Autodesk Fusion 360 part; units mm, degrees
(part 5 of 5)
sketch "Sketch2" plane through (0, 0, 2) normal (0, 0, 1) x (1, 0, 0)
  arc A0 (20.1662, -102.4349) -> (20.2, -101.6132) centre (10.2, -101.6132) ccw
  line L0 (20.2, -101.6132) -> (20.2, -87.2749)
  arc A1 (22.987, -85.4363) -> (20.2, -87.2749) centre (22.2, -87.2749) ccw
  line L1 (22.987, -85.4363) -> (27.3521, -87.3046)
  arc A2 (27.3521, -87.3046) -> (36.4601, -74.6136) centre (30.5, -79.95) ccw
  line L2 (36.4601, -74.6136) -> (31.6483, -69.2394)
  arc A3 (29.5877, -66.4969) -> (31.6483, -69.2394) centre (46.5487, -55.8985) ccw
  line L3 (29.5877, -66.4969) -> (23.2215, -56.3087)
  arc A4 (21.55, -50.4796) -> (23.2215, -56.3087) centre (32.55, -50.4796) ccw
  line L4 (21.55, -50.4796) -> (21.55, -18.7607)
  arc A5 (23.2215, -12.9316) -> (21.55, -18.7607) centre (32.55, -18.7607) ccw
  line L5 (23.2215, -12.9316) -> (27.7114, -5.7461)
  arc A6 (33.9547, -0.1656) -> (27.7114, -5.7461) centre (40.4322, -13.6949) ccw
  arc A7 (33.9547, -0.1656) -> (30.5, 15.05) centre (30.5, 7.05) ccw
  line L6 (30.5, 15.05) -> (9.313, 15.05)
  arc A8 (5, 18) -> (9.313, 15.05) centre (9.313, 19.6778) ccw
  line L7 (5, 18) -> (-5, 18)
  arc A9 (-9.313, 15.05) -> (-5, 18) centre (-9.313, 19.6778) ccw
  line L8 (-9.313, 15.05) -> (-30.5, 15.05)
  arc A10 (-30.5, 15.05) -> (-33.9547, -0.1656) centre (-30.5, 7.05) ccw
  arc A11 (-27.7114, -5.7461) -> (-33.9547, -0.1656) centre (-40.4322, -13.6949) ccw
  line L9 (-27.7114, -5.7461) -> (-23.2215, -12.9316)
  arc A12 (-21.55, -18.7607) -> (-23.2215, -12.9316) centre (-32.55, -18.7607) ccw
  line L10 (-21.55, -18.7607) -> (-21.55, -50.4796)
  arc A13 (-23.2215, -56.3087) -> (-21.55, -50.4796) centre (-32.55, -50.4796) ccw
  line L11 (-23.2215, -56.3087) -> (-29.5877, -66.4969)
  arc A14 (-31.6483, -69.2394) -> (-29.5877, -66.4969) centre (-46.5487, -55.8985) ccw
  line L12 (-31.6483, -69.2394) -> (-36.4601, -74.6136)
  arc A15 (-36.4601, -74.6136) -> (-27.3521, -87.3046) centre (-30.5, -79.95) ccw
  line L13 (-27.3521, -87.3046) -> (-22.987, -85.4363)
  arc A16 (-20.2, -87.2749) -> (-22.987, -85.4363) centre (-22.2, -87.2749) ccw
  line L14 (-20.2, -87.2749) -> (-20.2, -101.6132)
  arc A17 (-20.2, -101.6132) -> (-20.1662, -102.4349) centre (-10.2, -101.6132) ccw
  line L15 (-20.1662, -102.4349) -> (-19.6835, -108.2886)
  arc A18 (-19.6835, -108.2886) -> (-19.1143, -110.8871) centre (-9.7173, -107.4669) ccw
  line L16 (-19.1143, -110.8871) -> (-15.7286, -120.1891)
  arc A19 (-15.7286, -120.1891) -> (-7.0571, -119.3647) centre (-11.5, -118.65) ccw
  arc A20 (-3.1079, -116) -> (-7.0571, -119.3647) centre (-3.1079, -120) ccw
  line L17 (-3.1079, -116) -> (3.1079, -116)
  arc A21 (7.0571, -119.3647) -> (3.1079, -116) centre (3.1079, -120) ccw
  arc A22 (7.0571, -119.3647) -> (15.7286, -120.1891) centre (11.5, -118.65) ccw
  line L18 (15.7286, -120.1891) -> (19.1143, -110.8871)
  arc A23 (19.1143, -110.8871) -> (19.6835, -108.2886) centre (9.7173, -107.4669) ccw
  line L19 (19.6835, -108.2886) -> (20.1662, -102.4349)
  circle A24 centre (-15.25, -49.85) radius 1.5
  arc A25 (-13.5, 3) -> (-15.1961, -0.0598) centre (-13.5, 1) ccw
  line L20 (-13.5, 3) -> (-10.3384, 3)
  arc A26 (-6.0958, 1.2426) -> (-10.3384, 3) centre (-10.3384, -3) ccw
  line L21 (-6.0958, 1.2426) -> (-4.8532, 0)
  line L22 (-4.8532, 0) -> (4.8532, 0)
  line L23 (4.8532, 0) -> (6.0958, 1.2426)
  arc A27 (10.3384, 3) -> (6.0958, 1.2426) centre (10.3384, -3) ccw
  line L24 (10.3384, 3) -> (13.5, 3)
  arc A28 (15.1961, -0.0598) -> (13.5, 3) centre (13.5, 1) ccw
  line L25 (15.1961, -0.0598) -> (9.0119, -10.0491)
  spline S0 degree 5 poles (9.0119, -10.0491) (8.9382, -10.1683) (8.7794, -10.3902) (8.5077, -10.6735) (8.0875, -10.964) (7.4965, -11.2156) (6.9894, -11.3405) (6.5947, -11.3892) (6.3253, -11.4) (6.189, -11.4) knots 0 0 0 0 0 0 0.2 0.4 0.6 0.8 1 1 1 1 1 1
  line L26 (6.189, -11.4) -> (-6.189, -11.4)
  spline S1 degree 5 poles (-6.189, -11.4) (-6.3253, -11.4) (-6.5947, -11.3892) (-6.9894, -11.3405) (-7.4965, -11.2156) (-8.0875, -10.964) (-8.5077, -10.6735) (-8.7794, -10.3902) (-8.9382, -10.1683) (-9.0119, -10.0491) knots -1 -1 -1 -1 -1 -1 -0.8 -0.6 -0.4 -0.2 0 0 0 0 0 0
  line L27 (-9.0119, -10.0491) -> (-15.1961, -0.0598)
  circle A29 centre (15.25, -49.85) radius 1.5
  circle A30 centre (15.25, -19.35) radius 1.5
  circle A31 centre (-15.25, -19.35) radius 1.5
  circle A32 centre (-15.25, -63.85) radius 1.5
  circle A33 centre (-30.5, 7.05) radius 3.375
  circle A34 centre (15, -73.65) radius 1.5
  circle A35 centre (-15, -73.65) radius 1.5
  circle A36 centre (-10, -44.6) radius 1.5
  circle A37 centre (10, -44.6) radius 1.5
  circle A38 centre (10, -24.6) radius 1.5
  circle A39 centre (-10, -24.6) radius 1.5
  line L28 (5.45, -24.029) -> (5.45, -45.171)
  arc A40 (5.2981, -46.9075) -> (5.45, -45.171) centre (-4.55, -45.171) ccw
  line L29 (5.2981, -46.9075) -> (4.4577, -51.6736)
  arc A41 (3.4729, -52.5) -> (4.4577, -51.6736) centre (3.4729, -51.5) ccw
  line L30 (3.4729, -52.5) -> (-3.4729, -52.5)
  arc A42 (-4.4577, -51.6736) -> (-3.4729, -52.5) centre (-3.4729, -51.5) ccw
  line L31 (-4.4577, -51.6736) -> (-5.2981, -46.9075)
  arc A43 (-5.45, -45.171) -> (-5.2981, -46.9075) centre (4.55, -45.171) ccw
  line L32 (-5.45, -45.171) -> (-5.45, -24.029)
  arc A44 (-5.2981, -22.2925) -> (-5.45, -24.029) centre (4.55, -24.029) ccw
  line L33 (-5.2981, -22.2925) -> (-4.4577, -17.5264)
  arc A45 (-3.4729, -16.7) -> (-4.4577, -17.5264) centre (-3.4729, -17.7) ccw
  line L34 (-3.4729, -16.7) -> (3.4729, -16.7)
  arc A46 (4.4577, -17.5264) -> (3.4729, -16.7) centre (3.4729, -17.7) ccw
  line L35 (4.4577, -17.5264) -> (5.2981, -22.2925)
  arc A47 (5.45, -24.029) -> (5.2981, -22.2925) centre (-4.55, -24.029) ccw
  circle A48 centre (30.5, 7.05) radius 3.375
  circle A49 centre (-30.5, -79.95) radius 3.375
  circle A50 centre (15.25, -63.85) radius 1.5
  circle A51 centre (15.25, 8.95) radius 1.5
  circle A52 centre (-15.25, 8.95) radius 1.5
  arc A53 (4.5, -61) -> (8.3897, -57.7389) centre (6.3028, -59.2001) ccw
  line L36 (4.5, -61) -> (-4.5, -61)
  arc A54 (-8.3897, -57.7389) -> (-4.5, -61) centre (-6.3028, -59.2001) ccw
  line L37 (-8.3897, -57.7389) -> (-8.0447, -57.2462)
  arc A55 (-6.6112, -56.5) -> (-8.0447, -57.2462) centre (-6.6112, -58.25) ccw
  line L38 (-6.6112, -56.5) -> (6.6112, -56.5)
  arc A56 (8.0447, -57.2462) -> (6.6112, -56.5) centre (6.6112, -58.25) ccw
  line L39 (8.0447, -57.2462) -> (8.3897, -57.7389)
  circle A57 centre (30.5, -79.95) radius 3.375
  circle A58 centre (11.5, -118.65) radius 1.5
  circle A59 centre (15, -103.65) radius 1.5
  circle A60 centre (-11.5, -118.65) radius 1.5
  circle A61 centre (-15, -103.65) radius 1.5
  line L40 (0, -116) -> (0, -61) construction
  line L41 (-15, -103.65) -> (-5.1101, -103.65) construction
  circle A62 centre (-10, -103.65) radius 1
  circle A63 centre (-10, -103.65) radius 3
  line L42 (-2.5, -103.3105) -> (-2.5, -113.346)
  line L43 (-2.5, -113.346) -> (-11.1856, -107.81)
  line L44 (-11.1856, -107.81) -> (-11.1856, -106.4058)
  line L45 (-2.5, -103.3105) -> (-4.5464, -101.7117)
  line L46 (-7, -103.65) -> (-7, -103.4617)
  line L47 (-5.25, -101.7117) -> (-4.5464, -101.7117)
  arc A64 (-5.25, -101.7117) -> (-7, -103.4617) centre (-5.25, -103.4617) ccw
  line L48 (-10, -103.65) -> (-10, -83.65) construction
  circle A65 centre (-10, -83.65) radius 1
  circle A66 centre (-10, -83.65) radius 3
  line L49 (-2.5, -84.401) -> (-2.5, -94.9628)
  line L50 (-2.5, -84.401) -> (-5.6804, -81.9162)
  line L51 (-2.5, -84.401) -> (1.142, -84.401) construction
  line L52 (-5.6804, -81.9162) -> (-7.3512, -85.0584)
  line L53 (-9.532, -86.6133) -> (-9.532, -90.422)
  line L54 (-9.532, -90.422) -> (-2.5, -94.9628)
  line L55 (10, -103.65) -> (10, -83.65) construction
  line L56 (2.5, -103.3105) -> (4.5464, -101.7117)
  line L57 (2.5, -103.3105) -> (2.5, -113.346)
  circle A67 centre (10, -103.65) radius 3
  line L58 (2.5, -113.346) -> (11.1856, -107.81)
  circle A68 centre (15, -103.65) radius 1.5
  line L59 (15, -103.65) -> (5.1101, -103.65) construction
  line L60 (11.1856, -107.81) -> (11.1856, -106.4058)
  line L61 (7, -103.65) -> (7, -103.4617)
  circle A69 centre (10, -103.65) radius 1
  line L62 (5.25, -101.7117) -> (4.5464, -101.7117)
  arc A70 (7, -103.4617) -> (5.25, -101.7117) centre (5.25, -103.4617) ccw
  line L63 (9.532, -90.422) -> (2.5, -94.9628)
  line L64 (2.5, -84.401) -> (2.5, -94.9628)
  line L65 (5.6804, -81.9162) -> (7.3512, -85.0584)
  line L66 (2.5, -84.401) -> (-1.142, -84.401) construction
  line L67 (2.5, -84.401) -> (5.6804, -81.9162)
  line L68 (9.532, -86.6133) -> (9.532, -90.422)
  circle A71 centre (10, -83.65) radius 3
  circle A72 centre (10, -83.65) radius 1
  point P0 (10.2, -101.6132)
  point P1 (9.7173, -107.4669)
  dimension "d33" = 2
  dimension "d34" = 5
  dimension "d35" = 6
  dimension "d36" = 2.5
  dimension "d37" = 1.75
  dimension "d38" = 20
  dimension "d39" = 2
  dimension "d40" = 6
  dimension "d41" = 2.5
  dimension "d42" = 128
  dimension "d43" = 142
  dimension "d44" = 80
  constraint midpoint L17 L40.start
  constraint midpoint L36 L40.end
  constraint coincident A61.centre L41.start
  constraint perpendicular L14 L41
  constraint coincident L41 A62.centre
  constraint concentric A62 A63
  constraint parallel L40 L42
  constraint coincident A63 L44.end
  constraint vertical L44
  constraint coincident L41 L46.start
  constraint coincident A63 L46.start
  constraint tangent A63 L46
  constraint perpendicular L46 L47
  constraint tangent L47 A64
  constraint tangent L46 A64
  constraint coincident A62.centre A63.centre
  constraint perpendicular L41 L48
  constraint coincident L48.end A65.centre
  constraint concentric A65 A66
  constraint vertical L49
  constraint horizontal L51
  constraint coincident A66 L52.end
  constraint tangent A66 L52
  constraint coincident A66 L53.start
  constraint parallel L48 L53
  constraint symmetric A17.centre L40 P0
  constraint symmetric A18.centre L40 P1
  constraint symmetric A61 L40 A68
  constraint symmetric L40 A61.centre A59.centre
  constraint symmetric L40 L41.end L59.end
  constraint symmetric L40 A62 A69
  constraint symmetric L40 A63 A67
  constraint symmetric L40 L42.start L56.start
  constraint symmetric L40 L42.end L57.end
  constraint symmetric L40 L43.end L58.end
  constraint symmetric L40 L44.end L60.end
  constraint symmetric L40 L45.end L56.end
  constraint symmetric L40 L46.start L61.start
  constraint symmetric L40 L47.start L62.start
  constraint symmetric L40 L46.end L61.end
  constraint symmetric L40 A64 A70
  constraint symmetric L40 A62.centre L55.start
  constraint symmetric L40 L48.end L55.end
  constraint symmetric L40 A65 A72
  constraint symmetric L40 A66 A71
  constraint symmetric L40 L49.start L64.start
  constraint symmetric L40 L49.end L63.end
  constraint symmetric L40 L50.end L65.start
  constraint symmetric L40 L51.end L66.end
  constraint symmetric L40 L52.end L65.end
  constraint symmetric L40 L53.start L68.start
  constraint symmetric L40 L53.end L63.start
  measures "d33" diameter of A62
  measures "d34" distance of A61.centre A62.centre
  measures "d35" diameter of A63
  measures "d36" distance of L40 L42
  measures "d37" radius of A64
  measures "d38" distance of A62.centre L48.end
  measures "d39" diameter of A65
  measures "d40" diameter of A66
  measures "d41" distance of L40 L49
  measures "d42" angle of L42 L45
  measures "d43" angle of L50 L51
  measures "d44" angle of L50 L52
extrude "Extrude2" cut sketch "Sketch2" against normal blind 2 contours A62 | A63 L42 L43 L44 L45 L46 L47 A64 | A65 | A66 L49 L50 L52 L53 L54 | L56 L57 A67 L58 L60 L61 L62 A70 | A69 | L63 L64 L65 L67 L68 A71 | A72
fillet "Fillet6" radius 2 4 edges at (-5.6804, -81.9162, 1) (-2.5, -84.401, 1) (2.5, -84.401, 1) (5.6804, -81.9162, 1)
fillet "Fillet7" radius 1 4 edges at (-2.5, -94.9628, 1) (2.5, -94.9628, 1) (2.5, -113.346, 1) (-2.5, -113.346, 1)
fillet "Fillet8" radius 1.5 4 edges at (-4.5464, -101.7117, 1) (-2.5, -103.3105, 1) (4.5464, -101.7117, 1) (2.5, -103.3105, 1)
fillet "Fillet9" radius 1.5 4 edges at (-9.532, -90.422, 1) (-9.532, -86.6133, 1) (9.532, -90.422, 1) (9.532, -86.6133, 1)
fillet "Fillet10" radius 1.5 4 edges at (11.1856, -107.81, 1) (11.1856, -106.4058, 1) (-11.1856, -107.81, 1) (-11.1856, -106.4058, 1)
sketch "Sketch3" plane through (0, 0, 2) normal (0, 0, 1) x (1, 0, 0)
  circle A0 centre (10, -103.65) radius 1
  circle A1 centre (-10, -83.65) radius 1
  line L0 (-5.25, -101.7117) -> (-5.0629, -101.7117)
  arc A2 (-4.1394, -102.0297) -> (-5.0629, -101.7117) centre (-5.0629, -103.2117) ccw
  line L1 (-4.1394, -102.0297) -> (-3.0765, -102.8601)
  arc A3 (-2.5, -104.0421) -> (-3.0765, -102.8601) centre (-4, -104.0421) ccw
  line L2 (-2.5, -104.0421) -> (-2.5, -111.5227)
  arc A4 (-4.0375, -112.366) -> (-2.5, -111.5227) centre (-3.5, -111.5227) ccw
  line L3 (-4.0375, -112.366) -> (-9.1581, -109.1022)
  arc A5 (-8.9013, -106.4416) -> (-9.1581, -109.1022) centre (-8.3519, -107.8373) ccw
  arc A6 (-8.9013, -106.4416) -> (-7, -103.65) centre (-10, -103.65) ccw
  line L4 (-7, -103.65) -> (-7, -103.4617)
  arc A7 (-5.25, -101.7117) -> (-7, -103.4617) centre (-5.25, -103.4617) ccw
  line L5 (8.8457, -90.8652) -> (4.0425, -93.9668)
  arc A8 (2.5, -93.1267) -> (4.0425, -93.9668) centre (3.5, -93.1267) ccw
  line L6 (2.5, -93.1267) -> (2.5, -85.3765)
  arc A9 (3.2687, -83.8004) -> (2.5, -85.3765) centre (4.5, -85.3765) ccw
  line L7 (3.2687, -83.8004) -> (3.8022, -83.3836)
  arc A10 (6.7994, -84.0207) -> (3.8022, -83.3836) centre (5.0335, -84.9596) ccw
  line L8 (6.7994, -84.0207) -> (7.3512, -85.0584)
  arc A11 (7.3512, -85.0584) -> (8.688, -86.3479) centre (10, -83.65) ccw
  arc A12 (9.532, -87.6968) -> (8.688, -86.3479) centre (8.032, -87.6968) ccw
  line L9 (9.532, -87.6968) -> (9.532, -89.6051)
  arc A13 (8.8457, -90.8652) -> (9.532, -89.6051) centre (8.032, -89.6051) ccw
  arc A14 (9.1581, -109.1022) -> (8.9013, -106.4416) centre (8.3519, -107.8373) ccw
  line L10 (9.1581, -109.1022) -> (4.0375, -112.366)
  arc A15 (2.5, -111.5227) -> (4.0375, -112.366) centre (3.5, -111.5227) ccw
  line L11 (2.5, -111.5227) -> (2.5, -104.0421)
  arc A16 (3.0765, -102.8601) -> (2.5, -104.0421) centre (4, -104.0421) ccw
  line L12 (3.0765, -102.8601) -> (4.1394, -102.0297)
  arc A17 (5.0629, -101.7117) -> (4.1394, -102.0297) centre (5.0629, -103.2117) ccw
  line L13 (5.0629, -101.7117) -> (5.25, -101.7117)
  arc A18 (7, -103.4617) -> (5.25, -101.7117) centre (5.25, -103.4617) ccw
  line L14 (7, -103.4617) -> (7, -103.65)
  arc A19 (7, -103.65) -> (8.9013, -106.4416) centre (10, -103.65) ccw
  line L15 (-4.0425, -93.9668) -> (-8.8457, -90.8652)
  arc A20 (-9.532, -89.6051) -> (-8.8457, -90.8652) centre (-8.032, -89.6051) ccw
  line L16 (-9.532, -89.6051) -> (-9.532, -87.6968)
  arc A21 (-8.688, -86.3479) -> (-9.532, -87.6968) centre (-8.032, -87.6968) ccw
  arc A22 (-8.688, -86.3479) -> (-7.3512, -85.0584) centre (-10, -83.65) ccw
  line L17 (-7.3512, -85.0584) -> (-6.7994, -84.0207)
  arc A23 (-3.8022, -83.3836) -> (-6.7994, -84.0207) centre (-5.0335, -84.9596) ccw
  line L18 (-3.8022, -83.3836) -> (-3.2687, -83.8004)
  arc A24 (-2.5, -85.3765) -> (-3.2687, -83.8004) centre (-4.5, -85.3765) ccw
  line L19 (-2.5, -85.3765) -> (-2.5, -93.1267)
  arc A25 (-4.0425, -93.9668) -> (-2.5, -93.1267) centre (-3.5, -93.1267) ccw
  circle A26 centre (-10, -103.65) radius 1
  circle A27 centre (10, -83.65) radius 1
  arc A28 (20.1662, -102.4349) -> (20.2, -101.6132) centre (10.2, -101.6132) ccw
  line L20 (20.2, -101.6132) -> (20.2, -87.2749)
  arc A29 (22.987, -85.4363) -> (20.2, -87.2749) centre (22.2, -87.2749) ccw
  line L21 (22.987, -85.4363) -> (27.3521, -87.3046)
  arc A30 (27.3521, -87.3046) -> (36.4601, -74.6136) centre (30.5, -79.95) ccw
  line L22 (36.4601, -74.6136) -> (31.6483, -69.2394)
  arc A31 (29.5877, -66.4969) -> (31.6483, -69.2394) centre (46.5487, -55.8985) ccw
  line L23 (29.5877, -66.4969) -> (23.2215, -56.3087)
  arc A32 (21.55, -50.4796) -> (23.2215, -56.3087) centre (32.55, -50.4796) ccw
  line L24 (21.55, -50.4796) -> (21.55, -18.7607)
  arc A33 (23.2215, -12.9316) -> (21.55, -18.7607) centre (32.55, -18.7607) ccw
  line L25 (23.2215, -12.9316) -> (27.7114, -5.7461)
  arc A34 (33.9547, -0.1656) -> (27.7114, -5.7461) centre (40.4322, -13.6949) ccw
  arc A35 (33.9547, -0.1656) -> (30.5, 15.05) centre (30.5, 7.05) ccw
  line L26 (30.5, 15.05) -> (9.313, 15.05)
  arc A36 (5, 18) -> (9.313, 15.05) centre (9.313, 19.6778) ccw
  line L27 (5, 18) -> (-5, 18)
  arc A37 (-9.313, 15.05) -> (-5, 18) centre (-9.313, 19.6778) ccw
  line L28 (-9.313, 15.05) -> (-30.5, 15.05)
  arc A38 (-30.5, 15.05) -> (-33.9547, -0.1656) centre (-30.5, 7.05) ccw
  arc A39 (-27.7114, -5.7461) -> (-33.9547, -0.1656) centre (-40.4322, -13.6949) ccw
  line L29 (-27.7114, -5.7461) -> (-23.2215, -12.9316)
  arc A40 (-21.55, -18.7607) -> (-23.2215, -12.9316) centre (-32.55, -18.7607) ccw
  line L30 (-21.55, -18.7607) -> (-21.55, -50.4796)
  arc A41 (-23.2215, -56.3087) -> (-21.55, -50.4796) centre (-32.55, -50.4796) ccw
  line L31 (-23.2215, -56.3087) -> (-29.5877, -66.4969)
  arc A42 (-31.6483, -69.2394) -> (-29.5877, -66.4969) centre (-46.5487, -55.8985) ccw
  line L32 (-31.6483, -69.2394) -> (-36.4601, -74.6136)
  arc A43 (-36.4601, -74.6136) -> (-27.3521, -87.3046) centre (-30.5, -79.95) ccw
  line L33 (-27.3521, -87.3046) -> (-22.987, -85.4363)
  arc A44 (-20.2, -87.2749) -> (-22.987, -85.4363) centre (-22.2, -87.2749) ccw
  line L34 (-20.2, -87.2749) -> (-20.2, -101.6132)
  arc A45 (-20.2, -101.6132) -> (-20.1662, -102.4349) centre (-10.2, -101.6132) ccw
  line L35 (-20.1662, -102.4349) -> (-19.6835, -108.2886)
  arc A46 (-19.6835, -108.2886) -> (-19.1143, -110.8871) centre (-9.7173, -107.4669) ccw
  line L36 (-19.1143, -110.8871) -> (-15.7286, -120.1891)
  arc A47 (-15.7286, -120.1891) -> (-7.0571, -119.3647) centre (-11.5, -118.65) ccw
  arc A48 (-3.1079, -116) -> (-7.0571, -119.3647) centre (-3.1079, -120) ccw
  line L37 (-3.1079, -116) -> (3.1079, -116)
  arc A49 (7.0571, -119.3647) -> (3.1079, -116) centre (3.1079, -120) ccw
  arc A50 (7.0571, -119.3647) -> (15.7286, -120.1891) centre (11.5, -118.65) ccw
  line L38 (15.7286, -120.1891) -> (19.1143, -110.8871)
  arc A51 (19.1143, -110.8871) -> (19.6835, -108.2886) centre (9.7173, -107.4669) ccw
  line L39 (19.6835, -108.2886) -> (20.1662, -102.4349)
  circle A52 centre (-15.25, -49.85) radius 1.5
  arc A53 (-13.5, 3) -> (-15.1961, -0.0598) centre (-13.5, 1) ccw
  line L40 (-13.5, 3) -> (-10.3384, 3)
  arc A54 (-6.0958, 1.2426) -> (-10.3384, 3) centre (-10.3384, -3) ccw
  line L41 (-6.0958, 1.2426) -> (-4.8532, 0)
  line L42 (-4.8532, 0) -> (4.8532, 0)
  line L43 (4.8532, 0) -> (6.0958, 1.2426)
  arc A55 (10.3384, 3) -> (6.0958, 1.2426) centre (10.3384, -3) ccw
  line L44 (10.3384, 3) -> (13.5, 3)
  arc A56 (15.1961, -0.0598) -> (13.5, 3) centre (13.5, 1) ccw
  line L45 (15.1961, -0.0598) -> (9.0119, -10.0491)
  spline S0 degree 5 poles (9.0119, -10.0491) (8.9382, -10.1683) (8.7794, -10.3902) (8.5077, -10.6735) (8.0875, -10.964) (7.4965, -11.2156) (6.9894, -11.3405) (6.5947, -11.3892) (6.3253, -11.4) (6.189, -11.4) knots 0 0 0 0 0 0 0.2 0.4 0.6 0.8 1 1 1 1 1 1
  line L46 (6.189, -11.4) -> (-6.189, -11.4)
  spline S1 degree 5 poles (-6.189, -11.4) (-6.3253, -11.4) (-6.5947, -11.3892) (-6.9894, -11.3405) (-7.4965, -11.2156) (-8.0875, -10.964) (-8.5077, -10.6735) (-8.7794, -10.3902) (-8.9382, -10.1683) (-9.0119, -10.0491) knots -1 -1 -1 -1 -1 -1 -0.8 -0.6 -0.4 -0.2 0 0 0 0 0 0
  line L47 (-9.0119, -10.0491) -> (-15.1961, -0.0598)
  circle A57 centre (15.25, -49.85) radius 1.5
  circle A58 centre (15.25, -19.35) radius 1.5
  circle A59 centre (-15.25, -19.35) radius 1.5
  circle A60 centre (-15.25, -63.85) radius 1.5
  circle A61 centre (-30.5, 7.05) radius 3.375
  circle A62 centre (15, -73.65) radius 1.5
  circle A63 centre (-15, -73.65) radius 1.5
  circle A64 centre (-10, -44.6) radius 1.5
  circle A65 centre (10, -44.6) radius 1.5
  circle A66 centre (10, -24.6) radius 1.5
  circle A67 centre (-10, -24.6) radius 1.5
  line L48 (5.45, -24.029) -> (5.45, -45.171)
  arc A68 (5.2981, -46.9075) -> (5.45, -45.171) centre (-4.55, -45.171) ccw
  line L49 (5.2981, -46.9075) -> (4.4577, -51.6736)
  arc A69 (3.4729, -52.5) -> (4.4577, -51.6736) centre (3.4729, -51.5) ccw
  line L50 (3.4729, -52.5) -> (-3.4729, -52.5)
  arc A70 (-4.4577, -51.6736) -> (-3.4729, -52.5) centre (-3.4729, -51.5) ccw
  line L51 (-4.4577, -51.6736) -> (-5.2981, -46.9075)
  arc A71 (-5.45, -45.171) -> (-5.2981, -46.9075) centre (4.55, -45.171) ccw
  line L52 (-5.45, -45.171) -> (-5.45, -24.029)
  arc A72 (-5.2981, -22.2925) -> (-5.45, -24.029) centre (4.55, -24.029) ccw
  line L53 (-5.2981, -22.2925) -> (-4.4577, -17.5264)
  arc A73 (-3.4729, -16.7) -> (-4.4577, -17.5264) centre (-3.4729, -17.7) ccw
  line L54 (-3.4729, -16.7) -> (3.4729, -16.7)
  arc A74 (4.4577, -17.5264) -> (3.4729, -16.7) centre (3.4729, -17.7) ccw
  line L55 (4.4577, -17.5264) -> (5.2981, -22.2925)
  arc A75 (5.45, -24.029) -> (5.2981, -22.2925) centre (-4.55, -24.029) ccw
  circle A76 centre (30.5, 7.05) radius 3.375
  circle A77 centre (-30.5, -79.95) radius 3.375
  circle A78 centre (15.25, -63.85) radius 1.5
  circle A79 centre (15.25, 8.95) radius 1.5
  circle A80 centre (-15.25, 8.95) radius 1.5
  arc A81 (4.5, -61) -> (8.3897, -57.7389) centre (6.3028, -59.2001) ccw
  line L56 (4.5, -61) -> (-4.5, -61)
  arc A82 (-8.3897, -57.7389) -> (-4.5, -61) centre (-6.3028, -59.2001) ccw
  line L57 (-8.3897, -57.7389) -> (-8.0447, -57.2462)
  arc A83 (-6.6112, -56.5) -> (-8.0447, -57.2462) centre (-6.6112, -58.25) ccw
  line L58 (-6.6112, -56.5) -> (6.6112, -56.5)
  arc A84 (8.0447, -57.2462) -> (6.6112, -56.5) centre (6.6112, -58.25) ccw
  line L59 (8.0447, -57.2462) -> (8.3897, -57.7389)
  circle A85 centre (30.5, -79.95) radius 3.375
  circle A86 centre (11.5, -118.65) radius 1.5
  circle A87 centre (15, -103.65) radius 1.5
  circle A88 centre (-11.5, -118.65) radius 1.5
  circle A89 centre (-15, -103.65) radius 1.5
equation "d6 = 12.7 mm - 11.4 mm"
equation "d12 = ( 40.4 / 2 ) * 1 mm"
equation "d17 = ( 23 / 2 ) * 1 mm"
equation "d34 = 2.5 mm + 1 mm + 1.5 mm"

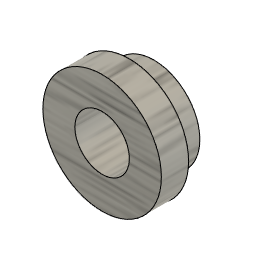
design "nut"
Autodesk Fusion 360 part; units mm, degrees
sketch "Sketch1" plane through (0, 0, 0) normal (0, 0, 1) x (1, 0, 0)
  circle A0 centre (0, 0) radius 4.35
  circle A1 centre (0, 0) radius 2
  dimension "d1" = 8.7
  dimension "d2" = 4
  constraint coincident A0.centre A1.centre
  measures "d1" diameter of A0
  measures "d2" diameter of A1
extrude "Extrude1" add sketch "Sketch1" along normal blind 2
sketch "Sketch2" plane through (0, 0, 0) normal (0, 0, -1) x (-1, 0, 0)
  circle A0 centre (0, 0) radius 2
  circle A1 centre (0, 0) radius 4.35
  circle A2 centre (0, 0) radius 2
  circle A3 centre (0, 0) radius 3.375
  dimension "d5" = 6.75
  constraint concentric A2 A3
  measures "d5" diameter of A3
extrude "Extrude2" add sketch "Sketch2" along normal blind 1.8 contours A3
